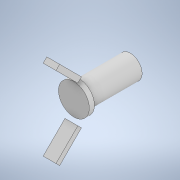
# Autodesk Inventor part: Weapon-Healing-Barrel
Saved by Autodesk Inventor 2020 (Build 240168000, 168)
## iProperties
Created: 2019-12-04
Part Number: Weapon-Healing-Barrel
Material: Generic
Document SubType Name: Modeling
Designer: Victor
Density: 1 g/cm^3
Appearance: Default
Author: Victor
Autodesk Inventor part; units mm, degrees
ref_plane "YZ Plane" through (0, 0, 0) normal (1, 0, 0) x (0, 1, 0)
ref_plane "XZ Plane" through (0, 0, 0) normal (0, 1, 0) x (-1, 0, 0)
ref_plane "XY Plane" through (0, 0, 0) normal (0, 0, 1) x (1, 0, 0)
sketch "Sketch1" plane through (0, 0, 0) normal (0, 0, 1) x (1, 0, 0)
  circle A0 centre (0, 0) radius 4.559
  dimension "d0" = 9.118
  constraints: 1 centre point, 1 coincident
  measures "d0" diameter of A0
extrude "Extrusion1" add sketch "Sketch1" along normal blind 20
sketch "Sketch3" plane through (0, 0, 20) normal (0, 0, 1) x (1, 0, 0)
  circle A0 centre (0, 0) radius 6
  dimension "d3" = 12
  constraints: 1 centre point, 1 coincident
  measures "d3" diameter of A0
extrude "Extrusion2" add sketch "Sketch3" along normal blind 2
sketch "Sketch4" plane through (0, 0, 0) normal (1, 0, 0) x (0, 1, 0)
  line L0 (7.1898, 22.9761) -> (15.6751, 31.4614)
  line L1 (7.1898, 22.9761) -> (19.1898, 22.9761) construction
  line L2 (15.6751, 31.4614) -> (17.0893, 30.0472)
  line L3 (17.0893, 30.0472) -> (8.604, 21.5619)
  line L4 (8.604, 21.5619) -> (7.1898, 22.9761)
  line L5 (6, 22) -> (-6, 22) projected
  line L6 (0, 36.5496) -> (0, 0)
  line L7 (-7.1898, 22.9761) -> (-15.6751, 31.4614)
  line L8 (-15.6751, 31.4614) -> (-17.0893, 30.0472)
  line L9 (-17.0893, 30.0472) -> (-8.604, 21.5619)
  line L10 (-8.604, 21.5619) -> (-7.1898, 22.9761)
  dimension "d6" = 12
  dimension "d7" = 45
  dimension "d8" = 2
  dimension "d9" = 0.9761
  dimension "d10" = 0.4381
  dimension "d11" = 2.604
  constraints: 20 end point, 4 symmetric about line, 2 perpendicular, 1 equal length, 1 horizontal, 1 vertical
  measures "d6" distance of L0.start L0.end
  measures "d7" angle of L1 L0
  measures "d8" distance of L0.end L2.end
  measures "d9" distance from line of L5 L0.start
  measures "d10" vertical distance of L5.start L3.end
  measures "d11" horizontal distance of L5.start L3.end
extrude "Extrusion3" add sketch "Sketch4" along normal mid plane 5
body "Solid1"
